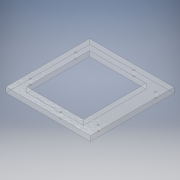
# Autodesk Inventor part: case_back_fix
Saved by Autodesk Inventor 2019 (Build 230136000, 136)
## iProperties
Created: 2019-02-02
Part Number: case_back_fix
Material: Acrylic, Clear
Document SubType Name: Modeling
Designer: suchanek
Density: 1.19 g/cm^3
Appearance: Transparent - Clear
Author: suchanek
Autodesk Inventor part; units mm, degrees
ref_plane "YZ Plane" through (0, 0, 0) normal (1, 0, 0) x (0, 1, 0)
ref_plane "XZ Plane" through (0, 0, 0) normal (0, 1, 0) x (-1, 0, 0)
ref_plane "XY Plane" through (0, 0, 0) normal (0, 0, 1) x (1, 0, 0)
sketch "Sketch1" plane through (0, 0, 0) normal (0, 1, 0) x (-1, 0, 0)
  line L0 (0, 0) -> (-5.6352, 0)
  line L1 (-5.6352, 0) -> (0, 0)
  line L2 (0, 0) -> (0, 8.7024)
  line L3 (0, -48) -> (97, -48)
  line L4 (97, -48) -> (97, 48)
  line L5 (97, 48) -> (0, 48)
  line L6 (0, 48) -> (0, -48)
  line L7 (85, -36) -> (20, -36)
  line L8 (20, -36) -> (20, 36)
  line L9 (20, 36) -> (85, 36)
  line L10 (85, 36) -> (85, -36)
  circle A0 centre (6, 33) radius 1.05
  circle A1 centre (6, -33) radius 1.05
  circle A2 centre (40, 42) radius 1.05
  circle A3 centre (91, 26) radius 1.05
  circle A4 centre (40, -42) radius 1.05
  circle A5 centre (91, -26) radius 1.05
  point P0 (0, -8.7024)
  dimension "d22" = 12
  dimension "d23" = 12
  dimension "d24" = 12
  dimension "d25" = 20
  dimension "d26" = 65
  dimension "d28" = 2.1
  dimension "d30" = 3
  dimension "d31" = 72
  dimension "d32" = 6
  dimension "d33" = 6
  dimension "d34" = 6
  dimension "d35" = 20
  dimension "d36" = 10
  constraints: 22 end point, 6 centre point, 5 equal length, 4 symmetric about line, 3 horizontal, 2 equal radius, 2 perpendicular, 1 midpoint, 1 vertical, 4 other
  measures "d22" distance between parallel lines of L10 L4
  measures "d23" distance between parallel lines of L5 L9
  measures "d24" distance between parallel lines of L3 L7
  measures "d25" distance between parallel lines of L8 L6
  measures "d26" distance between parallel lines of L8 L10
  measures "d28" diameter of A0
  measures "d30" distance from line of L9 A0.centre
  measures "d31" distance of L9.end L7.start
  measures "d32" distance from line of L6 A1.centre
  measures "d33" distance from line of L9 A2.centre
  measures "d34" distance from line of L10 A3.centre
  measures "d35" distance from line of L8 A4.centre
  measures "d36" distance from line of L7 A5.centre
extrude "Extrusion1" add sketch "Sketch1" along normal blind 6
equation "\"d22\" = d23"
equation "\"d24\" = d23"
body "Solid1"
